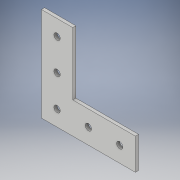
# Autodesk Inventor part: bracket
Saved by Autodesk Inventor 2018 (Build 220112000, 112)
## iProperties
Created: 2018-12-12
Part Number: bracket
Material: Generic
Document SubType Name: Modeling
Designer: s-4008082
Density: 1 g/cm^3
Appearance: Default
Author: s-4008082
Autodesk Inventor part; units mm, degrees
ref_plane "YZ Plane" through (0, 0, 0) normal (1, 0, 0) x (0, 1, 0)
ref_plane "XZ Plane" through (0, 0, 0) normal (0, 1, 0) x (-1, 0, 0)
ref_plane "XY Plane" through (0, 0, 0) normal (0, 0, 1) x (1, 0, 0)
sketch "Sketch1" plane through (0, 0, 0) normal (0, 0, 1) x (1, 0, 0)
  line L0 (0, 0) -> (-76.2, 0)
  line L1 (-76.2, 0) -> (-76.2, 25.4)
  line L2 (-76.2, 25.4) -> (0, 25.4)
  line L3 (0, 25.4) -> (0, 0)
  line L4 (-76.2, 25.4) -> (-50.8, 25.4)
  line L5 (-50.8, 25.4) -> (-50.8, 76.2)
  line L6 (-50.8, 76.2) -> (-76.2, 76.2)
  line L7 (-76.2, 76.2) -> (-76.2, 25.4)
  circle A0 centre (-63.5, 63.5) radius 2.5797
  circle A1 centre (-63.5, 38.1) radius 2.5797
  circle A2 centre (-63.5, 12.7) radius 2.5797
  circle A3 centre (-38.1, 12.7) radius 2.5797
  circle A4 centre (-12.7, 12.7) radius 2.5797
  dimension "d0" = 76.2
  dimension "d1" = 25.4
  dimension "d2" = 50.8
  dimension "d3" = 25.4
  dimension "d4" = 12.7
  dimension "d5" = 12.7
  dimension "d6" = 12.7
  dimension "d7" = 25.4
  dimension "d8" = 25.4
  dimension "d9" = 5.1594
  dimension "d10" = 5.1594
  dimension "d11" = 5.1594
  dimension "d12" = 5.1594
  dimension "d13" = 5.1594
  dimension "d14" = 12.7
  dimension "d15" = 25.4
  dimension "d16" = 12.7
  constraints: 16 end point, 5 centre point, 4 parallel, 2 horizontal, 2 perpendicular
  measures "d0" distance of L1.end L2.end
  measures "d1" distance of L2.end L0.start
  measures "d2" distance of L6.end L1.end
  measures "d3" distance of L5.end L6.end
  measures "d4" distance from line of L2 A4.centre
  measures "d5" distance from line of L3 A4.centre
  measures "d6" distance from line of L2 A3.centre
  measures "d7" distance of A4.centre A3.centre
  measures "d8" distance of A3.centre A2.centre
  measures "d9" diameter of A2
  measures "d10" diameter of A3
  measures "d11" diameter of A4
  measures "d12" diameter of A1
  measures "d13" diameter of A0
  measures "d14" distance from line of L5 A1.centre
  measures "d15" distance of A0.centre A1.centre
  measures "d16" distance from line of L6 A0.centre
extrude "Extrusion1" add sketch "Sketch1" along normal blind 2.54
body "Solid1"
